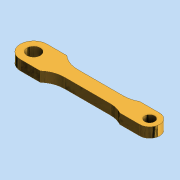
# Autodesk Inventor part: Connecting Rod
Saved by Autodesk Inventor 2018.2 (Build 222227000, 227)
## iProperties
Created: 2023-02-12
Part Number: Connecting Rod
Material: Generic
Document SubType Name: Modeling
Designer: NiveshandNisheeth
Density: 1 g/cm^3
Appearance: Brass - Satin
Author: NiveshandNisheeth
Autodesk Inventor part; units mm, degrees
ref_plane "YZ Plane" through (0, 0, 0) normal (1, 0, 0) x (0, 1, 0)
ref_plane "XZ Plane" through (0, 0, 0) normal (0, 1, 0) x (-1, 0, 0)
ref_plane "XY Plane" through (0, 0, 0) normal (0, 0, 1) x (1, 0, 0)
sketch "Sketch1" plane through (0, 0, 0) normal (0, 0, 1) x (1, 0, 0)
  line L0 (-17.5, 0) -> (17.5, 0) construction
  arc A0 (-17.5, 4) -> (-17.5, -4) centre (-17.5, 0) ccw
  arc A1 (17.5, -3) -> (17.5, 3) centre (17.5, 0) ccw
  circle A2 centre (-17.5, 0) radius 2
  circle A3 centre (17.5, 0) radius 1.5
  line L1 (-17.5, 4) -> (-11.5, 4)
  line L2 (17.5, 3) -> (11.5, 3)
  arc A4 (-11.5, 4) -> (-6.2085, 2) centre (-6.2085, 10) ccw
  arc A5 (7.627, 2) -> (11.5, 3) centre (7.627, 10) ccw
  line L3 (-6.2085, 2) -> (7.627, 2)
  line L4 (-17.5, -4) -> (-11.5, -4)
  line L5 (17.5, -3) -> (11.5, -3)
  arc A6 (-6.2085, -2) -> (-11.5, -4) centre (-6.2085, -10) ccw
  arc A7 (11.5, -3) -> (7.627, -2) centre (7.627, -10) ccw
  line L6 (-6.2085, -2) -> (7.627, -2)
  point P0 (0, 0)
  point P1 (0, 0)
  dimension "d0" = 35
  dimension "d1" = 8
  dimension "d2" = 6
  dimension "d3" = 4
  dimension "d4" = 3
  dimension "d5" = 6
  dimension "d6" = 8
  dimension "d7" = 2
  constraints: 16 end point, 12 point on circle, 8 centre point, 8 symmetric about line, 5 coincident, 4 horizontal, 4 tangent, 2 vertical alignment, 1 equal radius, 1 midpoint, 1 parallel, 2 other
  measures "d0" distance of L0.start L0.end
  measures "d1" diameter of A0
  measures "d2" diameter of A1
  measures "d3" diameter of A2
  measures "d4" diameter of A3
  measures "d5" distance of L1.start L1.end
  measures "d6" radius of A4
  measures "d7" distance between parallel lines of L0 L3
extrude "Extrusion1" add sketch "Sketch1" along normal mid plane 3
body "Solid1"
